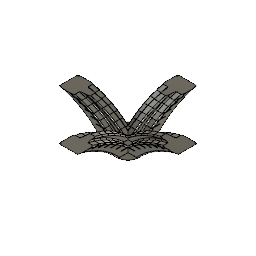
bear_overhang_45-75 (Autodesk Fusion 360 design; units mm, degrees)
Autodesk Fusion 360 part; units mm, degrees
sketch "arm" plane through (0, 0, 0) normal (0, 1, 0) x (1, 0, 0) in component "bear_overhang"
  line L0 (17.8, 0) -> (0, 0)
  line L1 (17.8, 0) -> (22, -4.2)
  line L2 (31.3844, -11.4) -> (36.5805, -14.4)
  line L3 (22, -4.2) -> (26.5287, -8)
  line L4 (26.5287, -8) -> (31.3844, -11.4)
  line L5 (0, -4.2) -> (0, 0)
  line L6 (8, -4.2) -> (0, -4.2)
  line L7 (0, 0) -> (0, -27.1786) construction
  line L8 (47.6512, -19) -> (33.6512, -19)
  line L9 (22.5805, -14.4) -> (17.3844, -11.4)
  line L10 (36.5805, -14.4) -> (22.5805, -14.4) construction
  line L11 (31.3844, -11.4) -> (17.3844, -11.4) construction
  line L12 (26.5287, -8) -> (12.5287, -8) construction
  line L13 (22, -4.2) -> (8, -4.2) construction
  line L14 (17.3844, -11.4) -> (12.5287, -8)
  line L15 (12.5287, -8) -> (8, -4.2)
  line L16 (8, -4.2) -> (3.8, 0)
  line L17 (14.5805, -14.4) -> (9.3844, -11.4)
  line L18 (9.3844, -11.4) -> (4.5287, -8)
  line L19 (4.5287, -8) -> (0, -4.2)
  line L20 (36.5805, -14.4) -> (42.1562, -17)
  line L21 (42.1562, -17) -> (47.6512, -19)
  line L22 (22.5805, -14.4) -> (28.1562, -17)
  line L23 (28.1562, -17) -> (33.6512, -19)
  line L24 (14.5805, -14.4) -> (20.1562, -17)
  line L25 (20.1562, -17) -> (25.6512, -19)
  line L26 (42.1562, -17) -> (28.1562, -17) construction
  line L27 (25.6512, -19) -> (31.6225, -20.6)
  line L28 (39.6225, -20.6) -> (53.6225, -20.6)
  line L29 (53.6225, -20.6) -> (47.6512, -19)
  line L30 (33.6512, -19) -> (39.6225, -20.6)
  line L31 (31.6225, -20.6) -> (39.6225, -20.6)
  dimension "d6" = 4.2
  dimension "d9" = 3.8
  dimension "d10" = 3.4
  dimension "d13" = 3
  dimension "d23" = 45
  dimension "d24" = 50
  dimension "d25" = 55
  dimension "d26" = 60
  dimension "d38" = 14
  dimension "d43" = 7.0711
  dimension "d44" = 7.5563
  dimension "d45" = 7.6
  dimension "d46" = 7.6019
  dimension "d50" = 65
  dimension "d51" = 70
  dimension "d52" = 2.6
  dimension "d53" = 2
  dimension "d54" = 6.6254
  dimension "d55" = 7.0171
  dimension "d77" = 75
  dimension "d78" = 8
  dimension "d79" = 14
  dimension "d80" = 1.6
  dimension "d81" = 9.5242
  constraint horizontal L8
  constraint horizontal L10
  constraint equal L8 L10
  constraint horizontal L11
  constraint equal L8 L11
  constraint equal L8 L12
  constraint equal L8 L13
  constraint horizontal L13
  constraint horizontal L12
  constraint coincident L0 L16.end
  constraint coincident L10 L17.start
  constraint horizontal L0
  constraint coincident L11 L17.end
  constraint coincident L12 L18.end
  constraint coincident L13 L5.start
  constraint parallel L15 L19
  constraint parallel L14 L18
  constraint parallel L9 L17
  constraint coincident L0.start L1.start
  constraint coincident L0.end L5.end
  constraint horizontal L26
  constraint equal L8 L26
  constraint parallel L22 L24
  constraint coincident L24.end L26
  constraint parallel L23 L25
  constraint perpendicular L0 L7
  constraint perpendicular L0 L5
  constraint equal L8 L28
  constraint parallel L28 L31
  constraint parallel L27 L30
  constraint coincident L8 L25.end
  measures "d6" distance of L1.end L0
  measures "d9" vertical distance of L3.end L1.end
  measures "d10" vertical distance of L3.end L2.start
  measures "d13" vertical distance of L2.end L2.start
  measures "d23" angle of L1 L7
  measures "d24" angle of L3 L7
  measures "d25" angle of L4 L7
  measures "d26" angle of L2 L7
  measures "d38" distance of L0.start L16.end
  measures "d50" angle of L7 L20
  measures "d51" angle of L7 L21
  measures "d52" vertical distance of L2.end L20.end
  measures "d53" vertical distance of L8.start L20.end
  measures "d77" angle of L7 L29
  measures "d78" distance of L28.start L27.end
  measures "d79" distance of L28.start L28.end
  measures "d80" distance of L8 L28
extrude "Extrude1" add sketch "arm" along normal mid plane 18 contours L0 L1 L2 L3 L4 L8 L9 L14 L15 L16 L20 L21 L22 L23 | L0 L5 L6 L16 | L8 L28 L29 L30 makes body 1 in component "bear_overhang"
extrude "Extrude2" add sketch "arm" along normal mid plane 6 contours L0 L5 L6 L16 | L6 L9 L14 L15 L17 L18 L19 L22 L23 L24 L25 L27 L30 L31 bodies 1 in component "bear_overhang"
fillet "Fillet1" radius 1 50 edges at (10.2643, -9, 6.1) (14.9565, -9, 9.7) (19.9824, -9, 12.9) (19.9, -9, 2.1) (24.2643, -9, 6.1) (28.9565, -9, 9.7) (33.9824, -9, 12.9) (10.2643, -3, 6.1) (14.9565, -3, 9.7) (19.9824, -3, 12.9) (33.9824, 9, 12.9) (28.9565, 9, 9.7) (24.2643, 9, 6.1) (19.9, 9, 2.1) (10.2643, 9, 6.1) (14.9565, 9, 9.7) (19.9824, 9, 12.9) (19.9824, 3, 12.9) (14.9565, 3, 9.7) (10.2643, 3, 6.1) (2.2643, 3, 6.1) (6.9565, 3, 9.7) (11.9824, 3, 12.9) (2.2643, -3, 6.1) (6.9565, -3, 9.7) (11.9824, -3, 12.9) (39.3684, -9, 15.7) (44.9037, -9, 18) (30.9037, -9, 18) (25.3684, -9, 15.7) (25.3684, -3, 15.7) (30.9037, -3, 18) (22.9037, -3, 18) (17.3684, -3, 15.7) (17.3684, 3, 15.7) (22.9037, 3, 18) (25.3684, 9, 15.7) (30.9037, 9, 18) (44.9037, 9, 18) (39.3684, 9, 15.7) (30.9037, 3, 18) (25.3684, 3, 15.7) (36.6368, 9, 19.8) (36.6368, 3, 19.8) (28.6368, 3, 19.8) (28.6368, -3, 19.8) (36.6368, -9, 19.8) (36.6368, -3, 19.8) (50.6368, 9, 19.8) (50.6368, -9, 19.8) on bodies 1 in component "bear_overhang"
sketch "angle_indication" plane through (0, -9, 0) normal (0, -1, 0) x (1, 0, 0) in component "bear_overhang"
  line L0 (22, 4.2) -> (8, 4.2)
  line L1 (26.5287, 8) -> (12.5287, 8)
  line L2 (31.3844, 11.4) -> (17.3844, 11.4)
  line L3 (36.5805, 14.4) -> (22.5805, 14.4)
  line L4 (42.1562, 17) -> (28.1562, 17)
  line L5 (8.2384, 4.4) -> (15.2384, 4.4)
  line L6 (15.2384, 4.4) -> (15, 4.2)
  line L7 (19.5287, 8) -> (19.8143, 8.2)
  line L8 (19.8143, 8.2) -> (12.8143, 8.2)
  line L9 (24.3844, 11.4) -> (24.7308, 11.6)
  line L10 (24.7308, 11.6) -> (17.7308, 11.6)
  line L11 (29.5805, 14.4) -> (30.0094, 14.6)
  line L12 (30.0094, 14.6) -> (23.0094, 14.6)
  line L13 (35.1562, 17) -> (35.7057, 17.2)
  line L14 (35.7057, 17.2) -> (28.7057, 17.2)
  line L15 (12.5287, 8) -> (8, 4.2)
  line L16 (17.3844, 11.4) -> (12.5287, 8)
  line L17 (22.5805, 14.4) -> (17.3844, 11.4)
  line L18 (28.1562, 17) -> (22.5805, 14.4)
  line L19 (33.6512, 19) -> (28.1562, 17)
  line L20 (39.6225, 20.6) -> (33.6512, 19)
  line L21 (33.6512, 19) -> (47.6512, 19)
  line L22 (34.3976, 19.2) -> (41.3976, 19.2)
  line L23 (41.3976, 19.2) -> (40.6512, 19)
  point P0 (22, 4.2)
  point P1 (26.5287, 8)
  point P2 (31.3844, 11.4)
  point P3 (36.5805, 14.4)
  point P4 (42.1562, 17)
  point P5 (47.6512, 19)
  dimension "d67" = 0.2
  dimension "d68" = 0.2
  dimension "d69" = 0.2
  dimension "d70" = 0.2
  dimension "d71" = 0.2
  dimension "d82" = 0.2
  constraint midpoint L0 L6.end
  constraint midpoint L1 L7.start
  constraint midpoint L2 L9.start
  constraint midpoint L3 L11.start
  constraint midpoint L4 L13.start
  constraint parallel L0 L5
  constraint parallel L1 L8
  constraint parallel L2 L10
  constraint parallel L3 L12
  constraint parallel L4 L14
  constraint coincident L14.end L19
  constraint coincident L4.end L18.start
  constraint coincident L3.end L17.start
  constraint coincident L2.end L16.start
  constraint coincident L1.end L15.start
  constraint coincident L5.start L15
  constraint coincident P0 L0.start
  constraint coincident P1 L1.start
  constraint coincident P2 L2.start
  constraint coincident P3 L3.start
  constraint coincident P4 L4.start
  constraint coincident L0.end L15.end
  constraint parallel L6 L15
  constraint parallel L7 L16
  constraint parallel L9 L17
  constraint parallel L11 L18
  constraint parallel L13 L19
  constraint coincident L12.end L18
  constraint coincident L10.end L17
  constraint coincident L8.end L16
  constraint coincident L19.start L20.end
  constraint coincident P5 L21.end
  constraint coincident L20 L22.start
  constraint parallel L21 L22
  constraint midpoint L21 L23.end
  constraint parallel L20 L23
  measures "d67" distance of L0 L5
  measures "d68" distance of L1 L8
  measures "d69" distance of L2 L10
  measures "d70" distance of L3 L12
  measures "d71" distance of L4 L14
  measures "d82" distance of L21 L22
extrude "Extrude2'" cut sketch "angle_indication" against normal blind 0.3 bodies 1 in component "bear_overhang"
mirror "Mirror1" about plane through (0, 0, 0) normal (0, 1, 0) of "Extrude2'" in component "bear_overhang"
pattern_circular "C-Pattern1" count 4 over 360 about axis through (0, 0, 1.75) along (0, 0, 1) of bodies 1 makes body 2 at (1.292, 45.9465, 20.6) makes body 3 at (-10.9239, 3, 0) makes body 4 at (3, -5.4619, 0) in component "bear_overhang"
combine "Combine1" operation add target body 1 tool bodies 2 3 4 in component "bear_overhang"
sketch "orientation_mark" plane through (0, 0, 0) normal (0, 0, -1) x (1, 0, 0) in component "bear_overhang"
  line L0 (-9, 9) -> (-16.3858, 9)
  ellipse E0 centre (-16.3858, 8) end of major axis (-17.8, 8) minor radius 1 (-16.3858, 9) -> (-17.8, 8) ccw
  line L1 (-17.8, 8) -> (-17.8, -8)
  ellipse E1 centre (-16.3858, -8) end of major axis (-17.8, -8) minor radius 1 (-17.8, -8) -> (-16.3858, -9) ccw
  line L2 (-16.3858, -9) -> (-9, -9)
  line L3 (-9, -9) -> (-9, -16.3858)
  ellipse E2 centre (-8, -16.3858) end of major axis (-8, -17.8) minor radius 1 (-9, -16.3858) -> (-8, -17.8) ccw
  line L4 (-8, -17.8) -> (8, -17.8)
  ellipse E3 centre (8, -16.3858) end of major axis (8, -17.8) minor radius 1 (8, -17.8) -> (9, -16.3858) ccw
  line L5 (9, -16.3858) -> (9, -9)
  line L6 (9, -9) -> (16.3858, -9)
  ellipse E4 centre (16.3858, -8) end of major axis (17.8, -8) minor radius 1 (16.3858, -9) -> (17.8, -8) ccw
  line L7 (17.8, -8) -> (17.8, 8)
  ellipse E5 centre (16.3858, 8) end of major axis (17.8, 8) minor radius 1 (17.8, 8) -> (16.3858, 9) ccw
  line L8 (16.3858, 9) -> (9, 9)
  line L9 (9, 9) -> (9, 16.3858)
  ellipse E6 centre (8, 16.3858) end of major axis (8, 17.8) minor radius 1 (9, 16.3858) -> (8, 17.8) ccw
  line L10 (8, 17.8) -> (-8, 17.8)
  ellipse E7 centre (-8, 16.3858) end of major axis (-8, 17.8) minor radius 1 (-8, 17.8) -> (-9, 16.3858) ccw
  line L11 (-9, 16.3858) -> (-9, 9)
  line L12 (-9, 9) -> (9, 9) construction
  line L13 (0, 9) -> (0, 17.8) construction
  circle A0 centre (0, 13.4) radius 1.5
  line L14 (-8, 17.8) -> (8, 17.8)
  line L15 (-17.8, -8) -> (-17.8, 8)
  line L16 (8, -17.8) -> (-8, -17.8)
  line L17 (17.8, 8) -> (17.8, -8)
  arc A1 (8, -17.8) -> (17.8, -8) centre (8, -8) ccw
  arc A2 (17.8, 8) -> (8, 17.8) centre (8, 8) ccw
  arc A3 (-8, 17.8) -> (-17.8, 8) centre (-8, 8) ccw
  arc A4 (-17.8, -8) -> (-8, -17.8) centre (-8, -8) ccw
  dimension "d56" = 3
  constraint coincident L0.start L11.end
  constraint coincident L8.end L9.start
  constraint midpoint L12 L13.start
  constraint midpoint L10 L13.end
  constraint midpoint L13 A0.centre
  constraint tangent L7 A1
  constraint coincident L7.start L17.end
  constraint coincident L4.end L16.start
  constraint tangent L10 A2
  constraint coincident L10.start L14.end
  constraint coincident L7.end L17.start
  constraint tangent L15 A3
  constraint coincident L1.start L15.end
  constraint coincident L10.end L14.start
  constraint tangent L16 A4
  constraint coincident L4.start L16.end
  constraint coincident L1.end L15.start
  measures "d56" diameter of A0
extrude "Extrude1'" cut sketch "orientation_mark" against normal blind 0.6 contours A0 bodies 1 in component "bear_overhang"
extrude "Extrude3" add sketch "orientation_mark" against normal blind 0.2 contours L0 E0 E7 L11 A3 | E1 L2 L3 E2 A4 | E5 L8 L9 E6 A2 | E3 L5 L6 E4 A1 bodies 1 in component "bear_overhang"
component "bear_overhang" placed x (1, 0, 0) y (0, 1, 0) z (0, 0, 1) at (0, 0, 0)
equation "d6 = layer_height * 21"
equation "d9 = layer_height * 19"
equation "d10 = layer_height * 17"
equation "d13 = layer_height * 15"
equation "d31 = arm_width"
equation "d34 = arm_support_width"
equation "d38 = arm_layer_length"
equation "layer_height = 0.2 mm"
equation "arm_width = 18 mm"
equation "arm_support_width = arm_width / 3"
equation "d52 = layer_height * 13"
equation "d53 = layer_height * 10"
equation "d57 = -layer_height * 3"
equation "arm_layer_length = 14 mm"
equation "d67 = layer_height"
equation "d68 = layer_height"
equation "d69 = layer_height"
equation "d70 = layer_height"
equation "d71 = layer_height"
equation "d75 = -layer_height"
equation "d78 = 22 mm - arm_layer_length"
equation "d79 = arm_layer_length"
equation "d80 = layer_height * 8"
equation "d82 = layer_height"
named bodies: "Body1 (1)"
